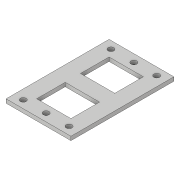
# Autodesk Inventor part: Part5
Saved by Autodesk Inventor 2018 (Build 220112000, 112)
## iProperties
Created: 2017-05-15
Part Number: Part5
Material: Generic
Document SubType Name: Modeling
Designer: anand
Density: 1 g/cm^3
Appearance: Default
Author: anand
Autodesk Inventor part; units mm, degrees
note: some values were not read from the file. Chosen so that the rebuilt part matches the saved one: pattern direction of "Rectangular Pattern1".
ref_plane "YZ Plane" through (0, 0, 0) normal (1, 0, 0) x (0, 1, 0)
ref_plane "XZ Plane" through (0, 0, 0) normal (0, 1, 0) x (-1, 0, 0)
ref_plane "XY Plane" through (0, 0, 0) normal (0, 0, 1) x (1, 0, 0)
sketch "Sketch1" plane through (0, 0, 0) normal (0, 1, 0) x (-1, 0, 0)
  line L0 (169.9997, 270) -> (-169.9997, 270)
  line L1 (-169.9997, 270) -> (-169.9997, -270)
  line L2 (-169.9997, -270) -> (169.9997, -270)
  line L3 (169.9997, -270) -> (169.9997, 270)
  line L4 (169.9997, 270) -> (-169.9997, -270) construction
  line L5 (-169.9997, 270) -> (169.9997, -270) construction
  point P0 (0, 0)
  dimension "d0" = 339.9993
  dimension "d1" = 539.9999
  constraints: 12 end point, 2 midpoint, 2 parallel, 1 horizontal, 1 perpendicular
  measures "d0" distance of L2.end L1.end
  measures "d1" distance of L0.end L1.end
extrude "Extrusion1" add sketch "Sketch1" along normal blind 20.0025
sketch "Sketch2" plane through (0, 20.0025, 0) normal (0, 1, 0) x (1, 0, 0)
  line L0 (-89.916, 189.8523) -> (89.916, 189.8523)
  line L1 (89.916, 189.8523) -> (89.916, 39.9923)
  line L2 (89.916, 39.9923) -> (-89.916, 39.9923)
  line L3 (-89.916, 39.9923) -> (-89.916, 189.8523)
  line L4 (-89.916, 189.8523) -> (89.916, 39.9923) construction
  line L5 (89.916, 189.8523) -> (-89.916, 39.9923) construction
  line L6 (-89.916, -39.9923) -> (89.916, -39.9923)
  line L7 (89.916, -39.9923) -> (89.916, -189.8523)
  line L8 (89.916, -189.8523) -> (-89.916, -189.8523)
  line L9 (-89.916, -189.8523) -> (-89.916, -39.9923)
  line L10 (-89.916, -39.9923) -> (89.916, -189.8523) construction
  line L11 (89.916, -39.9923) -> (-89.916, -189.8523) construction
  line L12 (-169.9997, -270) -> (169.9997, -270) projected
  line L13 (0, 0) -> (-323.2387, 0) construction
  point P0 (0, 114.9223)
  point P1 (0, -114.9223)
  point P2 (0, -114.9223)
  dimension "d4" = 149.86
  dimension "d5" = 149.86
  dimension "d6" = 179.832
  dimension "d7" = 179.832
  dimension "d9" = 79.9846
  constraints: 26 end point, 5 midpoint, 4 parallel, 3 horizontal, 2 perpendicular, 1 point on line, 1 vertical alignment, 1 other
  measures "d4" distance of L8.end L6.start
  measures "d5" distance of L2.end L0.start
  measures "d6" distance of L6.start L6.end
  measures "d7" distance of L0.start L0.end
  measures "d9" distance between parallel lines of L6 L2
extrude "Extrusion2" cut sketch "Sketch2" against normal through all
hole "Hole1" at (-119.9998, 20.0025, 229.995) direction (0, -1, 0) diameter 29.9999 end through all
pattern_linear "Rectangular Pattern1" count 2 spacing 459.994 along (0, 0, -1) count 3 spacing 119.9998 along (1, 0, 0) of "Hole1"
body "Solid1"
